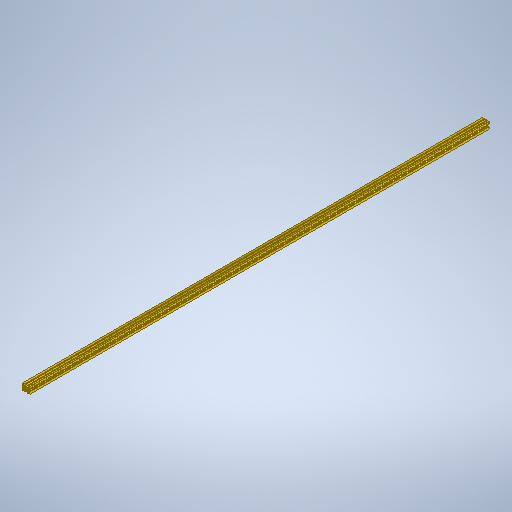
# Autodesk Inventor part: Perfil 30×30 2 rasgos adjacentes_AST03003002A
Saved by Autodesk Inventor 2025.2 (Build 292293000, 293)
## iProperties
Created: 2025-04-05
Part Number: Perfil 30×30 2 rasgos adjacentes_AST03003002A
Material: Ouro
Document SubType Name: Modeling
Designer: Gustavo Sousa
Density: 19.3 g/cm^3
Appearance: Metal quente 2400F
Author: Gustavo Sousa
Autodesk Inventor part; units mm, degrees
ref_plane "YZ Plane" through (0, 0, 0) normal (1, 0, 0) x (0, 1, 0)
ref_plane "XZ Plane" through (0, 0, 0) normal (0, 1, 0) x (-1, 0, 0)
ref_plane "XY Plane" through (0, 0, 0) normal (0, 0, 1) x (1, 0, 0)
sketch "Esboço1" plane through (0, 0, 0) normal (0, 0, 1) x (1, 0, 0)
  line L0 (-15, 15) -> (15, 15) construction
  line L1 (-15, -15) -> (15, -15) construction
  line L2 (-15, 15) -> (-15, -15) construction
  line L3 (15, 15) -> (15, -15) construction
  circle A0 centre (0, 0) radius 5
  line L4 (0, 0) -> (-15, 15) construction
  line L5 (15, 15) -> (0, 0) construction
  line L6 (-4.1, -15) -> (4.1, -15) construction
  line L7 (0, 0) -> (-15, -15) construction
  line L8 (0, 0) -> (15, -15) construction
  line L9 (-7, -7) -> (7, -7) construction
  line L10 (-7, 7) -> (-7, -7) construction
  line L11 (7, 7) -> (7, -7) construction
  line L12 (-7, 7) -> (7, 7) construction
  line L13 (-4.1, -15) -> (-4.6, -15) construction
  line L14 (-4.6, -15) -> (-4.6, -14.5)
  line L15 (-4.6, -14.5) -> (-4.1, -14.5)
  line L16 (-4.1, -14.5) -> (-4.1, -15) construction
  arc A1 (-15, -14.5) -> (-14.5, -15) centre (-14.5, -14.5) ccw
  line L17 (-14.5, -15) -> (-4.6, -15)
  line L18 (-4.1, -15) -> (-4.1, -12.8) construction
  line L19 (-4.1, -12.8) -> (-7.9, -12.8) construction
  line L20 (-5.4444, -7) -> (-7.9, -9.4556) construction
  line L21 (-7.9, -9.4556) -> (-7.9, -12.8) construction
  line L22 (-5.4444, -7) -> (0, -7) construction
  circle A2 centre (-11.5, -11.5) radius 2.5
  line L23 (-7, -5.4444) -> (-9.4556, -7.9) construction
  line L24 (-14, -7.9) -> (-9.4556, -7.9) construction
  line L25 (-7, -5.4444) -> (-7, 0) construction
  line L26 (-7, 0) -> (-7, 7) construction
  line L27 (-7, 7) -> (0, 7) construction
  circle A3 centre (-11.5, 11.5) radius 2.5 construction
  arc A4 (-14.5, 15) -> (-15, 14.5) centre (-14.5, 14.5) ccw
  line L28 (-15, 14.5) -> (-15, -14.5)
  line L29 (-14, -7.9) -> (-14, -6.6722) construction
  line L30 (-11.5, -11.5) -> (-14, -11.5) construction
  line L31 (-12.8, -4.2231) -> (-12.8, -6.6722)
  line L32 (-12.8, -6.6722) -> (-14, -6.6722)
  circle A5 centre (-3.5355, 3.5355) radius 1.1 construction
  line L33 (0, 0) -> (-3.5355, 3.5355) construction
  arc A6 (-2.6769, 4.2231) -> (-4.2231, 2.6769) centre (-3.5355, 3.5355) ccw
  arc A7 (-4.2231, -2.6769) -> (-2.6769, -4.2231) centre (-3.5355, -3.5355) ccw
  arc A8 (2.6769, -4.2231) -> (4.2231, -2.6769) centre (3.5355, -3.5355) ccw
  arc A9 (4.2231, 2.6769) -> (2.6769, 4.2231) centre (3.5355, 3.5355) ccw
  line L34 (-12.8, -4.2231) -> (-14, -4.2231)
  line L35 (-14, -4.2231) -> (-14, 2.6769)
  line L36 (-14, 2.6769) -> (-12.8, 2.6769)
  line L37 (-12.8, 2.6769) -> (-12.8, 5.126)
  line L38 (-14, 5.126) -> (-12.8, 5.126)
  line L39 (-14, 7.9) -> (-14, 5.126) construction
  line L40 (-11.5, 11.5) -> (-11.5, 9) construction
  line L41 (-14, 7.9) -> (-10.0913, 7.9) construction
  line L42 (-11.5, 11.5) -> (-7, 0) construction
  line L43 (-11.5, 11.5) -> (-10.589, 9.1719) construction
  line L44 (-10.589, 9.1719) -> (-10.0913, 7.9)
  line L45 (-11.5, 11.5) -> (0, 7) construction
  line L46 (-14.5, 15) -> (0, 15)
  line L47 (-11.5, 11.5) -> (-9.1719, 10.589) construction
  line L48 (-9.1719, 10.589) -> (-7.9, 10.0913) construction
  line L49 (-7.9, 14) -> (-7.9, 10.0913) construction
  arc A10 (-13.2678, 13.2678) -> (-10.589, 9.1719) centre (-11.5, 11.5) ccw
  arc A11 (-10.589, 9.1719) -> (-9.7322, 9.7322) centre (-11.5, 11.5) ccw
  line L50 (-13.2678, 13.2678) -> (-9.7322, 9.7322)
  line L51 (-9.7322, 9.7322) -> (-7, 7)
  line L52 (0, 7) -> (0, 5)
  line L53 (0, -7) -> (0, -5)
  line L54 (-13.2678, 13.2678) -> (-14.8536, 14.8536)
  arc A12 (14.5, -15) -> (15, -14.5) centre (14.5, -14.5) ccw
  line L55 (14.5, -15) -> (4.1, -15) construction
  line L56 (0, -7) -> (5.4444, -7) construction
  line L57 (4.1, -12.8) -> (4.1, -15) construction
  line L58 (-4.1, -14.5) -> (-4.1, -12.8)
  line L59 (4.1, -12.8) -> (7.9, -12.8) construction
  line L60 (7.9, -9.4556) -> (5.4444, -7) construction
  line L61 (7.9, -9.4556) -> (7.9, -12.8) construction
  circle A13 centre (11.5, -11.5) radius 2.5 construction
  arc A14 (9.7322, -9.7322) -> (13.2678, -13.2678) centre (11.5, -11.5) ccw
  line L62 (-7, 7) -> (9.7322, -9.7322)
  line L63 (13.2678, -13.2678) -> (14.8536, -14.8536)
  arc A15 (-13.5, 7.9) -> (-14, 7.4) centre (-13.5, 7.4) ccw
  line L64 (-14, 7.4) -> (-14, 5.126)
  arc A16 (-13.5, 7.9) -> (-10.0913, 7.9) centre (-11.7957, 10.7419) ccw
  arc A17 (-14, -7.4) -> (-13.5, -7.9) centre (-13.5, -7.4) ccw
  line L65 (-14, -6.6722) -> (-14, -7.4)
  arc A18 (-9.6627, -7.9) -> (-9.3092, -7.7536) centre (-9.6627, -7.4) ccw
  arc A19 (-7.1464, -5.5908) -> (-7, -5.2373) centre (-7.5, -5.2373) ccw
  arc A20 (-6.5, 7) -> (-7, 6.5) centre (-6.5, 6.5) ccw
  line L66 (-7, 6.5) -> (-7, -5.2373)
  line L67 (-7.1464, -5.5908) -> (-9.3092, -7.7536)
  line L68 (-9.6627, -7.9) -> (-13.5, -7.9)
  line L69 (-6.5, 7) -> (0, 7)
  arc A21 (-7.9, -12.3) -> (-7.4, -12.8) centre (-7.4, -12.3) ccw
  arc A22 (-7.7536, -9.3092) -> (-7.9, -9.6627) centre (-7.4, -9.6627) ccw
  arc A23 (-5.2373, -7) -> (-5.5908, -7.1464) centre (-5.2373, -7.5) ccw
  line L70 (-7.9, -9.6627) -> (-7.9, -12.3)
  line L71 (-7.4, -12.8) -> (-4.1, -12.8)
  line L72 (-7.7536, -9.3092) -> (-5.5908, -7.1464)
  arc A24 (5.5908, -7.1464) -> (5.2373, -7) centre (5.2373, -7.5) ccw
  arc A25 (7.9, -9.6627) -> (7.7536, -9.3092) centre (7.4, -9.6627) ccw
  arc A26 (7.4, -12.8) -> (7.9, -12.3) centre (7.4, -12.3) ccw
  line L73 (4.1, -12.8) -> (7.4, -12.8)
  line L74 (-5.2373, -7) -> (5.2373, -7)
  line L75 (5.5908, -7.1464) -> (7.7536, -9.3092)
  line L76 (7.9, -9.6627) -> (7.9, -12.3)
  line L77 (4.1, -15) -> (4.6, -15) construction
  line L78 (4.6, -15) -> (4.6, -14.5)
  line L79 (4.6, -14.5) -> (4.1, -14.5)
  line L80 (4.1, -14.5) -> (4.1, -15) construction
  line L81 (4.1, -12.8) -> (4.1, -14.5)
  line L82 (4.6, -15) -> (14.5, -15)
  point P0 (0, -15)
  point P1 (0, -15)
  point P2 (-8.2278, -6.6722)
  point P3 (-2.6769, -4.2231)
  point P4 (2.6769, -4.2231)
  point P5 (4.2231, -2.6769)
  point P6 (4.3134, -4.3134)
  point P7 (-4.3134, 4.3134)
  point P8 (3.5355, -3.5355)
  point P9 (-3.5355, 3.5355)
  point P10 (-6.8536, 6.8536)
  dimension "d19" = 5
  dimension "d0" = 30
  dimension "d5" = 30
  dimension "d6" = 15
  dimension "d7" = 10
  dimension "d8" = 8.2
  dimension "d9" = 8
  dimension "d11" = 2
  dimension "quadrado" = 0.5
  dimension "d13" = 0.5
  dimension "d23" = 1.1
  dimension "d26" = 11.5
  dimension "d27" = 2.2
  dimension "d28" = 1.1
  dimension "d29" = 1.1
  dimension "d33" = 2.2
  dimension "d34" = 2.2
  dimension "d37" = 360
  dimension "d39" = 1.1
  constraints: 166 end point, 60 point on circle, 44 point on line, 32 tangent, 26 centre point, 23 collinear, 17 equal length, 17 horizontal, 15 vertical, 13 equal radius, 7 midpoint, 7 parallel, 5 horizontal alignment, 5 vertical alignment, 4 coincident, 4 concentric, 4 perpendicular, 21 other
  measures "d0" distance of L0.start L0.end
  measures "d5" distance of L1.end L0.end
  measures "d6" distance from line of point (0, 0) L0
  measures "d7" diameter of A0
  measures "d8" distance of L6.start L6.end
  measures "d9" distance between parallel lines of L1 L9
  measures "d11" distance edge to line of A0 L12
  measures "quadrado" distance of L14.end L15.end
  measures "d13" radius of A1
  measures "d26" horizontal distance of L30.start point (0, 0)
  measures "d27" distance between parallel lines of L1 L19
  measures "d28" distance between parallel lines of L20 L7
  measures "d29" distance between parallel lines of L7 L23
  measures "d33" distance between parallel lines of L2 L31
  measures "d34" diameter of A5
  measures "d39" distance edge to line of A3 L41
extrude "Extrusão2" add sketch "Esboço1" along normal mid plane 2000 contours L62 A14 L63 A12 L82 L78 L79 L81 L73 A26 L76 A25 L75 A24 L74 L53 A0 A8 | L53 L74 A23 L72 A22 L70 A21 L71 L58 L15 L14 L17 A1 L28 A4 L54 A10 L44 A16 A15 L64 L38 L37 L36 L35 L34 L31 L32 L65 A17 L68 A18 L67 A19 L66 A20 L62 A6 A0 A7
mirror "Espelhar2" about plane through (-13.2678, 13.2678, 0) normal (0.7071068, 0.7071068, 0) of "Extrusão2"
equation "\"d23\" = 0.5 * espessura"
equation "\"d28\" = 0.5 * espessura"
equation "\"d29\" = 0.5 * espessura"
equation "\"espessura\" = 2.2"
